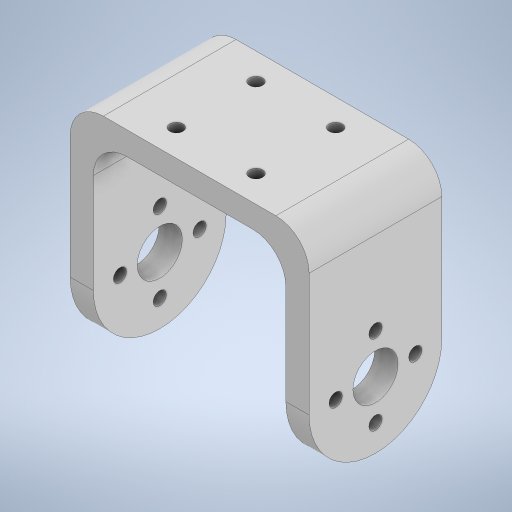
# Autodesk Inventor part: Motor_Bracket
Saved by Autodesk Inventor 2024 (Build 280153000, 153)
## iProperties
Created: 2024-06-01
Part Number: Motor_Bracket
Material: Generic
Document SubType Name: Modeling
Designer: Hemant
Density: 1 g/cm^3
Appearance: Default
Mass: 5.78849 g
Surface Area: 44.5118 cm^2
Volume: 5.78849 cm^3
Author: Hemant
Autodesk Inventor part; units mm, degrees
ref_plane "YZ Plane" through (0, 0, 0) normal (1, 0, 0) x (0, 1, 0)
ref_plane "XZ Plane" through (0, 0, 0) normal (0, 1, 0) x (-1, 0, 0)
ref_plane "XY Plane" through (0, 0, 0) normal (0, 0, 1) x (1, 0, 0)
sketch "Sketch1" plane through (0, 0, 0) normal (0, 0, 1) x (1, 0, 0)
  line L0 (14.5, -15) -> (-14.5, -15) construction
  line L1 (-14.5, -15) -> (-14.5, 15)
  line L2 (-14.5, 15) -> (14.5, 15)
  line L3 (14.5, 15) -> (14.5, -15)
  line L4 (14.5, -15) -> (-14.5, 15) construction
  line L5 (-14.5, -15) -> (14.5, 15) construction
  line L6 (-14.5, -15) -> (-18, -15)
  line L7 (-18, -15) -> (-18, 18.5)
  line L8 (-18, 18.5) -> (18, 18.5)
  line L9 (18, 18.5) -> (18, -15)
  line L10 (18, -15) -> (14.5, -15)
  point P0 (0, 0)
  dimension "d0" = 29
  dimension "d1" = 30
  dimension "d2" = 3.5
  dimension "d3" = 33.5
  dimension "d4" = 36
  constraints: 22 end point, 5 perpendicular, 2 midpoint, 2 parallel, 2 point on line, 1 horizontal
  measures "d0" distance of L1.end L2.end
  measures "d1" distance of L0.end L1.end
  measures "d2" distance of L0.end L6.end
  measures "d3" distance of L6.end L7.end
  measures "d4" distance of L7.end L8.end
extrude "Extrusion1" add sketch "Sketch1" along normal blind 20
sketch "Sketch2" plane through (-18, -15, 0) normal (-1, 0, 0) x (0, 0, 1)
  arc A0 (0, 10) -> (20, 10) centre (10, 10) ccw
  line L0 (20, 33.5) -> (20, 0) projected
  line L1 (0, 0) -> (20, 0) construction
  line L2 (0, 10) -> (0, 0)
  line L3 (0, 0) -> (20, 0) projected
  line L4 (0, 0) -> (20, 0)
  line L5 (20, 0) -> (20, 10)
  circle A1 centre (10, 10) radius 3.4
  circle A2 centre (10, 10) radius 6 construction
  circle A3 centre (4, 10) radius 1
  circle A4 centre (16, 10) radius 1
  circle A5 centre (10, 16) radius 1
  circle A6 centre (10, 4) radius 1
  point P0 (0, 15)
  point P1 (10, 0)
  dimension "d7" = 20
  dimension "d8" = 10
  dimension "d9" = 10
  dimension "d10" = 6.8
  dimension "d11" = 12
  dimension "d12" = 2
  dimension "d13" = 2
  dimension "d14" = 2
  dimension "d15" = 2
  constraints: 7 centre point, 6 end point, 6 point on circle, 2 coincident, 2 horizontal alignment, 2 vertical alignment, 1 horizontal, 1 point on line, 1 tangent
  measures "d7" diameter of A0
  measures "d8" distance from line of L0 A0.centre
  measures "d9" distance from line of L1 A0.centre
  measures "d10" diameter of A1
  measures "d11" diameter of A2
  measures "d12" diameter of A3
  measures "d13" diameter of A4
  measures "d14" diameter of A5
  measures "d15" diameter of A6
extrude "Extrusion2" cut sketch "Sketch2" against normal through all
fillet "Fillet1" radius 5 4 edges at (-14.5, 15, 10) (14.5, 15, 10) (-18, 18.5, 10) (18, 18.5, 10)
sketch "Sketch3" plane through (-9.5, 15, 0) normal (0, -1, 0) x (1, 0, 0)
  line L0 (-8.2697, 20) -> (0, 20) projected
  line L1 (0, 20) -> (19, 20) construction
  line L2 (19, 20) -> (27.2697, 20) projected
  line L3 (27.2697, 20) -> (27.2697, 0) projected
  line L4 (27.2697, 0) -> (19, 0) projected
  line L5 (19, 20) -> (19, 0) construction
  line L6 (-8.2697, 0) -> (-8.2697, 20) projected
  line L7 (0, 0) -> (-8.2697, 0) projected
  line L8 (0, 20) -> (0, 0) construction
  line L9 (19, 0) -> (0, 0) construction
  line L10 (3.5, 16) -> (15.5, 16) construction
  line L11 (15.5, 16) -> (15.5, 4) construction
  line L12 (15.5, 4) -> (3.5, 4) construction
  line L13 (3.5, 4) -> (3.5, 16) construction
  line L14 (3.5, 16) -> (15.5, 4) construction
  line L15 (15.5, 16) -> (3.5, 4) construction
  circle A0 centre (3.5, 16) radius 1
  circle A1 centre (15.5, 16) radius 1
  circle A2 centre (3.5, 4) radius 1
  circle A3 centre (15.5, 4) radius 1
  point P0 (9.5, 0)
  point P1 (9.5, 10)
  dimension "d19" = 12
  dimension "d20" = 12
  dimension "d21" = 10
  dimension "d22" = 9.5
  dimension "d23" = 2
  dimension "d24" = 2
  dimension "d25" = 2
  dimension "d26" = 2
  constraints: 12 end point, 4 centre point, 4 coincident, 2 midpoint, 2 parallel, 1 horizontal, 1 perpendicular
  measures "d19" distance of L11.end L12.end
  measures "d20" distance of L10.end L11.end
  measures "d21" distance from line of L9 point (9.5, 10)
  measures "d22" distance from line of L5 point (9.5, 10)
  measures "d23" diameter of A0
  measures "d24" diameter of A1
  measures "d25" diameter of A2
  measures "d26" diameter of A3
extrude "Extrusion3" cut sketch "Sketch3" against normal through all
sketch "Sketch4" plane through (-9.5, 15, 0) normal (0, -1, 0) x (1, 0, 0)
  circle A0 centre (3.5, 4) radius 1 construction
  circle A1 centre (15.5, 16) radius 1 construction
  circle A2 centre (15.5, 4) radius 1 construction
  circle A3 centre (3.5, 16) radius 1 construction
  line L0 (-8.2697, 20) -> (0, 20) projected
  line L1 (0, 20) -> (19, 20) construction
  line L2 (19, 20) -> (27.2697, 20) projected
  line L3 (27.2697, 20) -> (27.2697, 0) projected
  line L4 (27.2697, 0) -> (19, 0) projected
  line L5 (19, 20) -> (19, 0) construction
  line L6 (-8.2697, 0) -> (-8.2697, 20) projected
  line L7 (0, 0) -> (-8.2697, 0) projected
  line L8 (0, 20) -> (0, 0) construction
  line L9 (19, 0) -> (0, 0) construction
  circle A4 centre (3.5, 16) radius 2.25
  circle A5 centre (15.5, 16) radius 2.25
  circle A6 centre (15.5, 4) radius 2.25
  circle A7 centre (3.5, 4) radius 2.25
  point P0 (9.5, 0)
  dimension "d29" = 4.5
  dimension "d30" = 4.5
  dimension "d31" = 4.5
  dimension "d32" = 4.5
  constraints: 4 centre point, 4 coincident
  measures "d29" diameter of A4
  measures "d30" diameter of A5
  measures "d31" diameter of A6
  measures "d32" diameter of A7
extrude "Extrusion4" cut sketch "Sketch4" against normal blind 1
body "Solid1"
